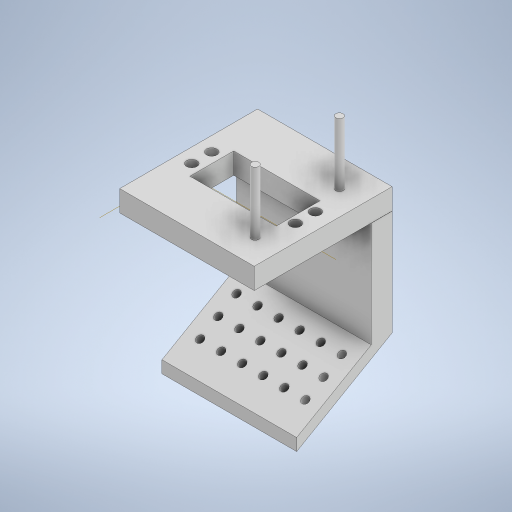
# Autodesk Inventor part: Part11
Saved by Autodesk Inventor 2024.1 (Build 281209000, 209)
## iProperties
Created: 2024-04-06
Part Number: Part11
Material: Generic
Document SubType Name: Modeling
Designer: elear
Density: 1 g/cm^3
Appearance: Default
Author: elear
Autodesk Inventor part; units mm, degrees
ref_plane "YZ Plane" through (0, 0, 0) normal (1, 0, 0) x (0, 1, 0)
ref_plane "XZ Plane" through (0, 0, 0) normal (0, 1, 0) x (-1, 0, 0)
ref_plane "XY Plane" through (0, 0, 0) normal (0, 0, 1) x (1, 0, 0)
sketch "Sketch1" plane through (0, 0, 0) normal (0, 1, 0) x (-1, 0, 0)
  circle A0 centre (-55, 20) radius 2.75
  circle A1 centre (-55, -20) radius 2.75
  circle A2 centre (-55, 20) radius 8
  circle A3 centre (-55, -20) radius 8
  circle A4 centre (-25.5769, 0) radius 21
  line L0 (-55.1769, 10.2) -> (-14.5769, 10.2)
  line L1 (-14.5769, 10.2) -> (-14.5769, -10.2)
  line L2 (-14.5769, -10.2) -> (-55.1769, -10.2)
  line L3 (-55.1769, -10.2) -> (-55.1769, 10.2)
  line L4 (-14.5769, 10.2) -> (-7.7769, 10.2)
  line L5 (-7.7769, 10.2) -> (-7.7769, -10.2)
  line L6 (-7.7769, -10.2) -> (-14.5769, -10.2)
  line L7 (-14.5769, -10.2) -> (-14.5769, 10.2)
  line L8 (-55.1769, 10.2) -> (-61.9769, 10.2)
  line L9 (-61.9769, 10.2) -> (-61.9769, -10.2)
  line L10 (-61.9769, -10.2) -> (-55.1769, -10.2)
  line L11 (-55.1769, -10.2) -> (-55.1769, 10.2)
  circle A5 centre (-9.5857, -4.75) radius 2.5
  circle A6 centre (-9.5857, 4.75) radius 2.5
  line L12 (-9.5857, 4.75) -> (-9.5857, -4.75)
  line L13 (-9.5857, -10.2) -> (-9.5857, -4.75)
  line L14 (-9.5857, 4.75) -> (-9.5857, 10.2)
  line L15 (-25.5769, 10.2) -> (-25.5769, 21)
  line L16 (-25.5769, -10.2) -> (-25.5769, -21)
  line L17 (-25.5769, 0) -> (-55.1769, 0)
  line L18 (13.335, 0) -> (-80.01, 0) projected
  line L19 (0, -46.4332) -> (0, 45.2366) projected
  line L20 (-4.5769, 0) -> (-7.7769, 0)
  circle A7 centre (-25.5769, 0) radius 18.1
  circle A8 centre (-55, 20) radius 6
  circle A9 centre (-55, -20) radius 5.6406
  circle A10 centre (-58.7982, -4.75) radius 2.5
  circle A11 centre (-58.7982, 4.75) radius 2.5
  line L21 (-2.7857, 32.1409) -> (-66.675, 32.1409)
  line L22 (-66.675, 32.1409) -> (-66.675, -33.3375)
  line L23 (-66.675, -33.3375) -> (-2.7857, -33.3375)
  line L24 (-2.7857, -33.3375) -> (-2.7857, 32.1409)
  line L25 (-6.1769, 12) -> (-63.8933, 12)
  line L26 (-63.8933, 12) -> (-63.8933, -12)
  line L27 (-63.8933, -12) -> (-6.1769, -12)
  line L28 (-6.1769, -12) -> (-6.1769, 12)
  circle A12 centre (-55, -20) radius 1.75
  circle A13 centre (-55, 20) radius 1.75
  line L29 (-49, 32.1409) -> (-49, 20)
  point P0 (0, 0)
  point P1 (-8.5769, -5.0781)
  dimension "d23" = 12
  dimension "d56" = -0.2
  dimension "d0" = 5.5
  dimension "d1" = 5.5
  dimension "d2" = 16
  dimension "d3" = 16
  dimension "d5" = 42
  dimension "d6" = 40.6
  dimension "d7" = 20.4
  dimension "d8" = 6.8
  dimension "d9" = 6.8
  dimension "d10" = 5
  dimension "d11" = 5
  dimension "d16" = 9.5
  dimension "d17" = 29.6
  dimension "d20" = -55
  dimension "d21" = -55
  dimension "d22" = 36.2
  dimension "d24" = 5
  dimension "d25" = 5
  dimension "d26" = 9.5
  dimension "d27" = 20
  dimension "d28" = 20
  dimension "d31" = 1
  constraints: 56 end point, 13 centre point, 12 point on line, 10 parallel, 8 coincident, 6 horizontal, 5 collinear, 5 perpendicular, 3 point on circle, 3 vertical, 2 midpoint, 1 equal radius, 1 horizontal alignment, 2 other
  measures "d0" diameter of A0
  measures "d1" diameter of A1
  measures "d2" diameter of A2
  measures "d3" diameter of A3
  measures "d5" diameter of A4
  measures "d6" distance of L0.start L0.end
  measures "d7" distance of L2.end L0.start
  measures "d8" distance between parallel lines of L1 L5
  measures "d9" distance between parallel lines of L9 L3
  measures "d10" diameter of A6
  measures "d11" diameter of A5
  measures "d16" distance of L12.start L12.end
  measures "d17" distance of L17.end L17.start
  measures "d20" distance from line of A1.centre L19
  measures "d21" distance from line of L19 A0.centre
  measures "d22" diameter of A7
  measures "d24" diameter of A11
  measures "d25" diameter of A10
  measures "d26" distance of A11.centre A10.centre
  measures "d27" distance from line of A2.centre L18
  measures "d28" distance from line of A1.centre L18
  measures "d31" radial gap between concentric circles of A12 A1
extrude "Extrusion1" add sketch "Sketch1" along normal blind 10 contours A0 | A1 | A2 | A2 L29 L21 L24 L18 A4 L28 L25 | A2 L25 L26 L18 L22 L21 L29 | L25 A4 L0 L8 L9 L18 L26 | L25 A7 L0 A4 | A4 L15 A7 L25 | A4 L25 A7 L15 | L25 L15 L0 A7 | A7 L15 L25 | A3 | L26 L27 A4 L28 L18 L24 L23 L22 | L18 L9 L10 L2 A4 L27 L26 | L25 L28 A4 | A4 L28 L18 A7 A6 L5 L4 L25 | A7 L25 L15 | L3 L18 L9 L8 | L25 A7 L4 L0 L15 | L18 L3 L10 L9 | L18 L28 A4 | A4 L28 L18 | L2 A7 L27 A4 | L28 L27 A4 | A4 L27 A7 L6 L5 A5 L18 L28 | A7 L14 A6 L12 L18 L1 L4 | L4 L14 A7 | L27 A7 L16 A4 | L2 L16 L27 A7 | A4 L16 A7 L27 | A7 A5 L5 L18 | L18 L5 A6 A7 | L4 L5 A6 A7 L14 | A7 A6 L14 | L27 L16 A7 | L2 L6 A7 L27 L16 | L18 L12 A5 L13 A7 L6 L1 | A7 L16 L27 | L18 L12 A6 L5 | L5 A5 L12 L18 | A7 L13 L6 | L13 A7 A5 L5 L6 | L13 A5 A7 | A8 | A9 | A12 | A13
extrude "Extrusion2" add sketch "Sketch1" along normal blind 30 from surface at 10 contours A12 | A13
move faces "Move5" translate (0, 0, 0.2) faces at (41.6436, 6.6667, 10.2)
move faces "Move6" translate (0, 0, -0.2) faces at (28.1103, 6.6667, -10.2)
move faces "Move7" translate (0.2, 0, 0) faces at (55.1769, 3.3333, -3.4667)
move faces "Move8" translate (-0.2, 0, 0) faces at (14.5769, 3.3333, 3.4667)
sketch "Sketch2" plane through (2.7857, 0, -33.3375) normal (-1, 0, 0) x (0, 0, 1)
  line L0 (0, 0) -> (0, 10) projected
  line L1 (55.5625, 0) -> (55.5625, -40.2602)
  line L2 (0, 0) -> (65.4784, 0) projected
  line L3 (23.8125, 0) -> (23.8125, -55)
  line L4 (0, 0) -> (10, 0)
  line L5 (10, 0) -> (10, -50)
  line L6 (10, -50) -> (0, -50)
  line L7 (0, -50) -> (0, 0)
  line L8 (10, -50) -> (45.3991, -70.4377)
  line L9 (45.3991, -70.4377) -> (45.3991, -76.2112)
  line L10 (45.3991, -76.2112) -> (0, -50)
  line L11 (26.0875, 10) -> (26.0875, 0) projected
  line L12 (65.4784, 0) -> (65.4784, 10) projected
  line L13 (0, 10) -> (65.4784, 10) projected
  line L14 (0, 0) -> (65.4784, 0) projected
  line L15 (65.4784, 0) -> (65.4784, 10) projected
  line L16 (0, 10) -> (65.4784, 10) projected
  line L17 (0, 0) -> (0, 10) projected
  line L18 (35.5875, 0) -> (40.5875, 0) projected
  line L19 (26.0875, 10) -> (31.0875, 10) projected
  line L20 (26.0875, 0) -> (31.0875, 0) projected
  line L21 (26.0875, 0) -> (31.0875, 0) projected
  line L22 (43.7375, 0) -> (22.9375, 0) projected
  line L23 (22.9375, 0) -> (22.9375, 10) projected
  line L24 (43.7375, 10) -> (22.9375, 10) projected
  line L25 (43.7375, 0) -> (43.7375, 10) projected
  line L26 (43.7375, 0) -> (22.9375, 0) projected
  line L27 (22.9375, 0) -> (22.9375, 10) projected
  line L28 (43.7375, 10) -> (22.9375, 10) projected
  line L29 (43.7375, 0) -> (43.7375, 10) projected
  line L30 (65.4784, 0) -> (65.4784, 10) projected
  line L31 (65.4784, 0) -> (65.4784, 10) projected
  line L32 (65.4784, 0) -> (65.4784, 10) projected
  line L33 (51.5875, 10) -> (55.0875, 10) projected
  line L34 (11.5875, 10) -> (15.0875, 10) projected
  line L35 (65.4784, 10) -> (0, 10) projected
  line L36 (0, 10) -> (65.4784, 10) projected
  line L37 (35.5875, 10) -> (40.5875, 10) projected
  line L38 (43.7375, 10) -> (22.9375, 10) projected
  line L39 (22.9375, 10) -> (43.7375, 10) projected
  line L40 (35.5875, 10) -> (40.5875, 10) projected
  line L41 (26.0875, 10) -> (31.0875, 10) projected
  line L42 (26.0875, 10) -> (31.0875, 10) projected
  line L43 (0, 0) -> (65.4784, 0) projected
  line L44 (65.4784, 0) -> (0, 0) projected
  line L45 (35.5875, 0) -> (40.5875, 0) projected
  line L46 (43.7375, 0) -> (22.9375, 0) projected
  line L47 (22.9375, 0) -> (43.7375, 0) projected
  line L48 (35.5875, 0) -> (40.5875, 0) projected
  line L49 (26.0875, 0) -> (31.0875, 0) projected
  line L50 (26.0875, 0) -> (31.0875, 0) projected
  line L51 (65.4784, 10) -> (0, 10) projected
  line L52 (65.4784, 0) -> (0, 0) projected
  line L53 (0, 0) -> (0, 10) projected
  line L54 (65.4784, 10) -> (0, 10) projected
  line L55 (65.4784, 0) -> (65.4784, 10) projected
  line L56 (65.4784, 0) -> (0, 0) projected
  line L57 (51.5875, 10) -> (55.0875, 10) projected
  line L58 (43.7375, 0) -> (43.7375, 10) projected
  line L59 (43.7375, 0) -> (43.7375, 10) projected
  line L60 (0, 0) -> (0, 10) projected
  line L61 (0, 0) -> (0, 10) projected
  line L62 (0, 0) -> (0, 10) projected
  line L63 (22.9375, 0) -> (22.9375, 10) projected
  line L64 (22.9375, 0) -> (22.9375, 10) projected
  line L65 (26.0875, 10) -> (31.0875, 10) projected
  line L66 (26.0875, 0) -> (31.0875, 0) projected
  line L67 (43.7375, 0) -> (43.7375, 10) projected
  line L68 (22.9375, 0) -> (22.9375, 10) projected
  line L69 (22.9375, 0) -> (43.7375, 0) projected
  line L70 (22.9375, 0) -> (43.7375, 0) projected
  line L71 (43.7375, 0) -> (43.7375, 10) projected
  line L72 (22.9375, 10) -> (43.7375, 10) projected
  line L73 (22.9375, 0) -> (22.9375, 10) projected
  line L74 (35.5875, 10) -> (40.5875, 10) projected
  line L75 (35.5875, 10) -> (40.5875, 10) projected
  line L76 (35.5875, 0) -> (40.5875, 0) projected
  line L77 (22.9375, 10) -> (43.7375, 10) projected
  line L78 (26.0875, 10) -> (31.0875, 10) projected
  line L79 (51.5875, 10) -> (55.0875, 10) projected
  line L80 (51.5875, 40) -> (55.0875, 40) projected
  line L81 (51.5875, 40) -> (55.0875, 40) projected
  line L82 (51.5875, 40) -> (55.0875, 40) projected
  line L83 (35.5875, 10) -> (40.5875, 10) projected
  line L84 (35.5875, 0) -> (40.5875, 0) projected
  line L85 (35.5875, 10) -> (40.5875, 10) projected
  line L86 (26.0875, 10) -> (31.0875, 10) projected
  line L87 (35.5875, 0) -> (40.5875, 0) projected
  line L88 (26.0875, 0) -> (31.0875, 0) projected
  line L89 (11.5875, 10) -> (15.0875, 10) projected
  line L90 (11.5875, 40) -> (15.0875, 40) projected
  line L91 (11.5875, 40) -> (15.0875, 40) projected
  line L92 (11.5875, 10) -> (15.0875, 10) projected
  line L93 (11.5875, 40) -> (15.0875, 40) projected
  line L94 (-13.0957, 0) -> (78.5741, 0) projected
  point P0 (33.3375, 0)
  point P1 (10, 0)
  dimension "d63" = 55
  dimension "d64" = 10
  dimension "d65" = 120
  dimension "d66" = 120
  dimension "d102" = 50
  constraints: 18 end point, 2 parallel, 2 perpendicular, 2 vertical, 1 horizontal, 15 other
  measures "d63" distance of L3.start L3.end
  measures "d64" distance between parallel lines of L5 L7
  measures "d65" angle of L5 L8
  measures "d66" angle of L7 L10
  measures "d102" distance of L6.end L0.start
extrude "Extrusion3" add sketch "Sketch2" against normal blind 65.5625 contours L2 L5 L6 L7 | L6 L8 L9 L10
move faces "Move9" translate (-1.588, 0, 0) faces at (68.3482, -16.6667, -30.0042) (27.9459, 0, 24.8939)
sketch "Sketch3" plane through (2.7857, -50, -33.3375) normal (0, -0.8660254, -0.5) x (1, 0, 0)
  circle A0 centre (57, 36.7033) radius 1.75
  circle A1 centre (47, 36.7033) radius 1.75
  circle A2 centre (37, 36.7033) radius 1.75
  line L0 (57, 36.7033) -> (47, 36.7033)
  line L1 (37, 36.7033) -> (47, 36.7033)
  circle A3 centre (57, 26.7033) radius 1.75
  circle A4 centre (47, 26.7033) radius 1.75
  circle A5 centre (37, 26.7033) radius 1.75
  line L2 (57, 26.7033) -> (47, 26.7033)
  line L3 (37, 26.7033) -> (47, 26.7033)
  circle A6 centre (57, 16.7033) radius 1.75
  circle A7 centre (47, 16.7033) radius 1.75
  circle A8 centre (37, 16.7033) radius 1.75
  line L4 (57, 16.7033) -> (47, 16.7033)
  line L5 (37, 16.7033) -> (47, 16.7033)
  circle A9 centre (27, 16.7033) radius 1.75
  circle A10 centre (17, 16.7033) radius 1.75
  circle A11 centre (7, 16.7033) radius 1.75
  line L6 (27, 16.7033) -> (17, 16.7033)
  line L7 (7, 16.7033) -> (17, 16.7033)
  circle A12 centre (27, 36.7033) radius 1.75
  circle A13 centre (17, 36.7033) radius 1.75
  circle A14 centre (7, 36.7033) radius 1.75
  line L8 (27, 36.7033) -> (17, 36.7033)
  line L9 (7, 36.7033) -> (17, 36.7033)
  circle A15 centre (27, 26.7033) radius 1.75
  circle A16 centre (17, 26.7033) radius 1.75
  circle A17 centre (7, 26.7033) radius 1.75
  line L10 (27, 26.7033) -> (17, 26.7033)
  line L11 (7, 26.7033) -> (17, 26.7033)
  line L12 (58.75, 36.7033) -> (64.329, 36.7033)
  line L13 (0, 49.5356) -> (0, 8.6603) projected
  line L14 (0, 36.7033) -> (7, 36.7033)
  point P0 (-2.7857, 3.8711)
  dimension "d72" = 3.5
  dimension "d73" = 10
  dimension "d74" = 3.5
  dimension "d75" = 10
  dimension "d76" = 0
  dimension "d77" = 10
  dimension "d78" = 3.5
  dimension "d79" = 10
  dimension "d84" = 3.5
  dimension "d85" = 10
  dimension "d90" = 3.5
  dimension "d91" = 10
  dimension "d92" = 3.5
  dimension "d93" = 10
  dimension "d94" = 0
  dimension "d95" = 10
  dimension "d96" = 10
  dimension "d97" = 10
  dimension "d98" = 10
  dimension "d101" = 7
  constraints: 28 end point, 17 centre point, 12 collinear, 11 equal radius, 7 horizontal, 1 horizontal alignment, 1 perpendicular, 1 point on line, 3 other
  measures "d73" distance of L0.start L0.end
  measures "d74" diameter of A3
  measures "d75" distance of L2.start L2.end
  measures "d76" horizontal distance of L1.start L3.start
  measures "d77" distance between parallel lines of L0 L2
  measures "d78" diameter of A6
  measures "d79" distance of L4.start L4.end
  measures "d84" diameter of A9
  measures "d85" distance of L6.start L6.end
  measures "d90" diameter of A12
  measures "d91" distance of L8.start L8.end
  measures "d92" diameter of A15
  measures "d93" distance of L10.start L10.end
  measures "d94" horizontal distance of L9.start L11.start
  measures "d95" distance between parallel lines of L8 L10
  measures "d96" distance of L2.start L4.start
  measures "d97" distance of L10.start L6.start
  measures "d98" distance of L10.start L3.start
  measures "d101" distance of L14.start L9.start
extrude "Extrusion4" cut sketch "Sketch3" against normal blind 30
body "Solid1"
